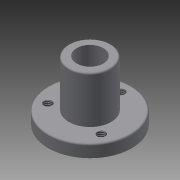
# Autodesk Inventor part: lead carriage
Saved by Autodesk Inventor 2015 (Build 190159000, 159)
## iProperties
Created: 2015-01-29
Part Number: lead carriage
Material: Generic
Document SubType Name: Modeling
Designer: Joseph
Density: 1 g/cm^3
Appearance: Default
Author: Joseph
Autodesk Inventor part; units mm, degrees
ref_plane "YZ Plane" through (0, 0, 0) normal (1, 0, 0) x (0, 1, 0)
ref_plane "XZ Plane" through (0, 0, 0) normal (0, 1, 0) x (-1, 0, 0)
ref_plane "XY Plane" through (0, 0, 0) normal (0, 0, 1) x (1, 0, 0)
sketch "Sketch1" plane through (0, 0, 0) normal (0, 0, 1) x (1, 0, 0)
  circle A0 centre (0, 0) radius 12.5
  dimension "d0" = 25
  constraints: 1 centre point, 1 coincident
  measures "d0" diameter of A0
extrude "Extrusion1" add sketch "Sketch1" along normal blind 3.75
sketch "Sketch2" plane through (0, 0, 3.75) normal (0, 0, 1) x (1, 0, 0)
  circle A0 centre (0, 0) radius 12.5 projected
  circle A1 centre (0, 0) radius 6.35
  dimension "d3" = 12.7
  constraints: 1 centre point, 1 coincident
  measures "d3" diameter of A1
extrude "Extrusion2" add sketch "Sketch2" along normal blind 14 contours A1
sketch "Sketch3" plane through (0, 0, 17.75) normal (0, 0, 1) x (1, 0, 0)
  circle A0 centre (0, 0) radius 6.35 projected
  constraints: 1 coincident
hole "Hole1" at (0, 0, 17.75) direction (0, 0, -1) diameter 8 end through all
sketch "Sketch4" plane through (0, 0, 3.75) normal (0, 0, 1) x (1, 0, 0)
  circle A0 centre (0, 0) radius 12.5 projected
  line L0 (-7.9971, -4.6239) -> (-0.0058, 9.2376) construction
  line L1 (-0.0058, 9.2376) -> (8.0029, -4.6137) construction
  line L2 (8.0029, -4.6137) -> (-7.9971, -4.6239) construction
  circle A1 centre (0, 0) radius 9.2376 construction
  dimension "d13" = 16
  constraints: 6 end point, 4 coincident, 3 point on circle, 2 equal length, 1 centre point
  measures "d13" distance of L0.start L0.end
hole "Hole2" at (-7.9971, -4.6239, 3.75) at (-0.0058, 9.2376, 3.75) at (8.0029, -4.6137, 3.75) direction (0, 0, -1) diameter 2.459 end through all thread size "M3x0.5" class "6H" standard "ANSI Metric M Profile"
fillet "Fillet1" radius 0.5 2 edges at (-12.5, 0, 3.75) (-6.35, 0, 17.75)
body "Solid1"
